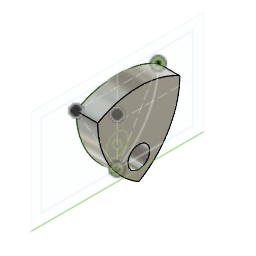
ruleaux (Autodesk Fusion 360 design; units mm, degrees)
part number: 2026-06-01-21-01-21-214
Autodesk Fusion 360 part; units mm, degrees
sketch "Excentric Triunghiular Ruleaux + Frame-ul cadrului culisant" plane through (0, 0, 0) normal (1, 0, 0) x (0, 1, 0)
  line L0 (-9.5, 5.4848) -> (0, -10.9697) construction
  line L1 (0, -10.9697) -> (9.5, 5.4848) construction
  line L2 (9.5, 5.4848) -> (-9.5, 5.4848) construction
  arc A0 (0, -10.9697) -> (9.5, 5.4848) centre (-9.5, 5.4848) ccw
  arc A1 (-9.5, 5.4848) -> (0, -10.9697) centre (9.5, 5.4848) ccw
  arc A2 (9.5, 5.4848) -> (-9.5, 5.4848) centre (0, -10.9697) ccw
  circle A3 centre (0, -6) radius 2.5
  line L3 (-17.5, 8.0303) -> (17.5, 8.0303)
  line L4 (17.5, 8.0303) -> (17.5, -10.9697)
  line L5 (17.5, -10.9697) -> (-17.5, -10.9697)
  line L6 (-17.5, -10.9697) -> (-17.5, 8.0303)
  line L7 (0, 8.0303) -> (0, -10.9697) construction
  line L8 (20, -13.4697) -> (-20, -13.4697)
  line L9 (-20, -13.4697) -> (-20, 10.5303)
  line L10 (-20, 10.5303) -> (20, 10.5303)
  line L11 (20, 10.5303) -> (20, -13.4697)
  line L12 (17.5, -1.4697) -> (0, -1.4697) construction
  dimension "d4" = 19
  dimension "d5" = 5
  dimension "d6" = 35
  dimension "d7" = 19
  dimension "d8" = 6
  dimension "d9" = 17.5
  dimension "d10" = -2.5
  constraint coincident L0.start L2.end
  constraint coincident L0.end L1.start
  constraint coincident L0.start A2
  constraint coincident L1.end L2.start
  constraint coincident L0.end A1
  constraint horizontal L3
  constraint vertical L4
  constraint horizontal L5
  constraint vertical L6
  constraint midpoint A2 L7.start
  constraint perpendicular L5 L7
  constraint midpoint L4 L12.start
  constraint midpoint L7 L12.end
  measures "d4" distance of L0.start L1.end
  measures "d5" diameter of A3
  measures "d6" distance of L3.start L3.end
  measures "d7" distance of L3.start L5.end
  measures "d8" distance of origin A3.centre
  measures "d9" distance of L4 L7
extrude "Extrude1" add sketch "Excentric Triunghiular Ruleaux + Frame-ul cadrului culisant" along normal blind 5 contours A0 A1 A2
equation "d9 = ( 35 / 2 ) * 1 mm"
named bodies: "Excentric Triunghiular Ruleaux"
